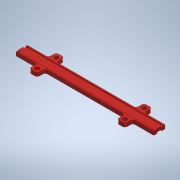
# Autodesk Inventor part: LED_Strip_Halter
Saved by Autodesk Inventor 2021.2 (Build 252289000, 289)
## iProperties
Part Number: LED_Strip_Halter
Material: PA 6 schwarz
Document SubType Name: Modeling
Designer: SRORF
Mass: 18.0608 g
Surface Area: 90.5069 cm^2
Volume: 15.8428 cm^3
Density: 1.14 g/cm^3
Appearance: Orangerot
ROT_Density: 1.0
PDB_Ident_Ver: =<PDB_Ident> <PDB_Version>
ROT_Weight: 0.018 kg
ROT_Weight_Num: 0.018060761989733748
Author: SRORF
Autodesk Inventor part; units mm, degrees
note: some values were not read from the file. Chosen so that the rebuilt part matches the saved one: pattern direction of "Rechteckige Anordnung2".
ref_plane "YZ Plane" through (0, 0, 0) normal (1, 0, 0) x (0, 1, 0)
ref_plane "XZ Plane" through (0, 0, 0) normal (0, 1, 0) x (-1, 0, 0)
ref_plane "XY Plane" through (0, 0, 0) normal (0, 0, 1) x (1, 0, 0)
sketch "Skizze2" plane through (0, 0, 0) normal (0, 0, 1) x (1, 0, 0)
  line L0 (-86.25, 7) -> (86.25, 7)
  line L1 (86.25, 7) -> (86.25, -7)
  line L2 (86.25, -7) -> (-86.25, -7)
  line L3 (-86.25, -7) -> (-86.25, 7)
  line L4 (0, 9.8) -> (0, -9.8) projected
  line L5 (-120.75, 0) -> (120.75, 0) projected
  point P0 (0, 0)
  point P1 (-86.25, 0)
  point P2 (0, 7)
  dimension "d0" = 14
  dimension "d1" = 172.5
  constraints: 8 end point, 2 midpoint, 2 parallel, 2 point on line, 1 horizontal, 1 perpendicular
  measures "d0" distance of L2.end L0.start
  measures "d1" distance of L0.start L0.end
extrude "Extrusion1" add sketch "Skizze2" along normal blind 3.5
sketch "Skizze3" plane through (0, 0, 3.5) normal (0, 0, 1) x (1, 0, 0)
  line L0 (86.25, -7) -> (86.25, 7) projected
  line L1 (86.25, 7) -> (-86.25, 7) projected
  line L2 (-86.25, 7) -> (-86.25, -7) projected
  line L3 (-86.25, -7) -> (86.25, -7) projected
  line L4 (86.25, 7) -> (-86.25, 7)
  line L5 (-86.25, 7) -> (-86.25, 5.5)
  line L6 (-86.25, 5.5) -> (86.25, 5.5)
  line L7 (86.25, 5.5) -> (86.25, 7)
  line L8 (-86.25, 7) -> (-86.25, -7) projected
  line L9 (-86.25, -7) -> (86.25, -7)
  line L10 (86.25, -7) -> (86.25, -5.5)
  line L11 (86.25, -5.5) -> (-86.25, -5.5)
  line L12 (-86.25, -5.5) -> (-86.25, -7)
  point P0 (0, 0)
  dimension "d4" = 1.5
  dimension "d5" = 1.5
  constraints: 16 end point, 4 parallel, 2 horizontal, 2 perpendicular, 2 point on line
  measures "d4" distance between parallel lines of L3 L11
  measures "d5" distance between parallel lines of L1 L6
extrude "Extrusion2" add sketch "Skizze3" along normal blind 1 contours L3 L2 L11 L0 | L6 L2 L1 L0
sketch "Skizze4" plane through (0, 0, 0) normal (0, 0, -1) x (-1, 0, 0)
  line L0 (86.25, -7) -> (-86.25, -7) projected
  line L1 (155.9309, -7) -> (147.0048, -7)
  line L2 (60, -7) -> (50, -7)
  line L3 (50, -7) -> (50, -17)
  line L4 (50, -17) -> (60, -17)
  line L5 (60, -17) -> (60, -7)
  line L6 (50, 7) -> (60, 7)
  line L7 (60, 7) -> (60, 17)
  line L8 (60, 17) -> (50, 17)
  line L9 (50, 17) -> (50, 7)
  line L10 (86.25, -7) -> (-86.25, -7) projected
  line L11 (-86.25, 7) -> (86.25, 7) projected
  line L12 (86.25, 7) -> (86.25, -7) projected
  line L13 (-60, -9.0118) -> (-60, -17) construction
  line L14 (-60, -17) -> (-50, -17) construction
  line L15 (-50, -17) -> (-50, -7) construction
  line L16 (-86.25, -7) -> (-86.25, 7) projected
  point P0 (0, 0)
  point P1 (50, -7)
  point P2 (55, -17)
  point P3 (-55, -17)
  point P4 (55, -12)
  point P5 (55, 12)
  point P6 (60, -12)
  point P7 (60, 12)
  dimension "d8" = 10
  dimension "d9" = 10
  dimension "d30" = 110
  dimension "d31" = 10
  dimension "d32" = 24
  dimension "d33" = 55
  constraints: 24 end point, 6 point on line, 5 parallel, 4 midpoint, 3 horizontal, 2 collinear, 2 horizontal alignment, 2 perpendicular, 2 vertical alignment, 1 vertical
  measures "d8" distance between parallel lines of L0 L4
  measures "d9" distance of L8.end L6.start
  measures "d30" distance of point (-55, -17) point (55, -17)
  measures "d31" distance of L3.end L4.end
  measures "d32" distance of point (55, -12) point (55, 12)
  measures "d33" horizontal distance of point (0, 0) point (55, -12)
extrude "Extrusion3" add sketch "Skizze4" against normal up to surface (4.5 mm away) contours L5 L4 L3 L0 | L6 L9 L8 L7
sketch "Skizze5" plane through (0, 0, 0) normal (0, 0, -1) x (-1, 0, 0)
  line L0 (50, -17) -> (60, -17) projected
  line L1 (50, -7) -> (50, -17) projected
  line L2 (50, 17) -> (50, 7) projected
  point P0 (0, 0)
  point P1 (55, -12)
  point P2 (55, 12)
  point P3 (55, -17)
  point P4 (50, -12)
  point P5 (50, 12)
  dimension "d13" = 24
  constraints: 3 midpoint, 2 horizontal alignment, 2 vertical alignment
  measures "d13" distance of point (55, -12) point (55, 12)
hole "Bohrung1" at (-55, -12, 0) direction (0, 0, 1) diameter 5.2 end through all
fillet "Rundung1" radius 3 8 edges at (-60, -17, 2.25) (-50, -17, 2.25) (-50, -7, 2.25) (-60, -7, 2.25) (-50, 17, 2.25) (-60, 17, 2.25) (-50, 7, 2.25) (-60, 7, 2.25)
pattern_linear "Rechteckige Anordnung1" count 2 spacing 24 along (0, 1, 0) of "Bohrung1"
pattern_linear "Rechteckige Anordnung2" count 2 spacing 110 along (1, 0, 0) of "Rundung1", "Bohrung1", "Extrusion3", "Rechteckige Anordnung1"
sketch "Skizze7" plane through (0, 0, 3.5) normal (0, 0, 1) x (1, 0, 0)
  line L0 (-86.25, 5.5) -> (-86.25, -5.5) projected
  line L1 (-86.25, 3) -> (-87.75, 3)
  line L2 (-87.75, 3) -> (-87.75, -3)
  line L3 (-87.75, -3) -> (-86.25, -3)
  line L4 (-86.25, -3) -> (-86.25, 3)
  line L5 (86.25, -3.1) -> (84.65, -3.1)
  line L6 (84.65, -3.1) -> (84.65, 3.1)
  line L7 (84.65, 3.1) -> (86.25, 3.1)
  line L8 (86.25, 3.1) -> (86.25, -3.1)
  line L9 (86.25, -5.5) -> (86.25, 5.5) projected
  point P0 (0, 0)
  point P1 (-87.75, 0)
  point P2 (-86.25, 0)
  point P3 (-86.25, 0)
  point P4 (84.65, 0)
  point P5 (86.25, 0)
  point P6 (86.25, 0)
  dimension "d37" = 1.5
  dimension "d38" = 6
  dimension "d41" = 1.6
  dimension "d44" = 6.2
  constraints: 16 end point, 6 midpoint, 4 parallel, 3 horizontal alignment, 2 horizontal, 2 perpendicular, 1 coincident, 1 collinear, 1 point on line
  measures "d37" distance between parallel lines of L0 L2
  measures "d38" distance of L1.end L2.end
  measures "d41" distance of L6.end L7.end
  measures "d44" distance of L5.end L6.end
extrude "Extrusion5" add sketch "Skizze7" against normal up to surface (3.5 mm away) contours L0 L3 L2 L1
extrude "Extrusion6" cut sketch "Skizze7" against normal through all contours L5 L6 L7 L8
equation "\"d5\" = d4"
equation "\"d9\" = d8"
equation "\"d33\" = 0.5 * d30"
equation "\"d24\" = d13"
